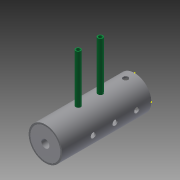
# Autodesk Inventor part: collector
Saved by Autodesk Inventor 2015 (Build 190159000, 159)
## iProperties
Created: 2014-11-05
Part Number: collector
Material: Generic
Document SubType Name: Modeling
Designer: lethcoec
Density: 1 g/cm^3
Appearance: Default
Author: lethcoec
Autodesk Inventor part; units mm, degrees
sketch "Sketch1" plane through (0, 0, 0) normal (0, 0, 1) x (1, 0, 0)
  circle A0 centre (0, 0) radius 19.05
  dimension "d0" = 38.1
  constraints: 1 centre point, 1 coincident
  measures "d0" diameter of A0
extrude "Extrusion1" add sketch "Sketch1" along normal blind 101.6
ref_plane "Work Plane1" through (19.05, 0, 0) normal (1, 0, 0) x (0, 1, 0)
sketch "Sketch3" plane through (19.05, 0, 0) normal (1, 0, 0) x (0, 1, 0)
  point P0 (0, 0)
sketch "Sketch4" plane through (19.05, 0, 0) normal (1, 0, 0) x (0, 1, 0)
  line L0 (0, 13.614358) -> (0, 19.507158)
  circle A0 centre (0, 16.560758) radius 2.9464
  point P0 (0, 0)
  dimension "d6" = 5.8928
  constraints: 2 end point, 1 midpoint, 1 vertical, 1 vertical alignment, 2 other
  measures "d6" distance of L0.start L0.end
hole "Hole1" at (19.05, 0, 16.560758) direction (-1, 0, 0) diameter 5.8928 end through all
sketch "Sketch5" plane through (19.05, 0, 0) normal (1, 0, 0) x (0, 1, 0)
  line L0 (0, 19.507155) -> (0, 38.353955)
  line L1 (0, 38.353955) -> (0, 44.246755)
  circle A0 centre (0, 41.300355) radius 2.9464
  point P0 (0, 0)
  dimension "d14" = 18.8468
  dimension "d15" = 5.8928
  constraints: 4 end point, 2 vertical, 1 midpoint, 1 vertical alignment, 2 other
  measures "d14" distance of L0.start L0.end
  measures "d15" distance of L0.end L1.end
hole "Hole2" at (19.05, 0, 41.300355) direction (-1, 0, 0) diameter 5.8928 end through all
sketch "Sketch6" plane through (19.05, 0, 0) normal (1, 0, 0) x (0, 1, 0)
  line L0 (0, 44.246748) -> (0, 63.093548)
  line L1 (0, 63.093548) -> (0, 68.986348)
  circle A0 centre (0, 66.039948) radius 2.9464
  point P0 (0, 0)
  dimension "d23" = 18.8468
  dimension "d24" = 5.8928
  constraints: 4 end point, 2 vertical, 1 midpoint, 1 vertical alignment, 2 other
  measures "d23" distance of L0.start L0.end
  measures "d24" distance of L0.end L1.end
hole "Hole3" at (19.05, 0, 66.039948) direction (-1, 0, 0) diameter 5.8928 end through all
sketch "Sketch7" plane through (0, 0, 0) normal (0, 0, -1) x (-1, 0, 0)
  circle A0 centre (0, 0) radius 19.05 projected
ref_plane "Work Plane2" through (0, 19.05, 0) normal (0, 1, 0) x (-1, 0, 0)
sketch "Sketch8" plane through (0, 19.05, 0) normal (0, 1, 0) x (-1, 0, 0)
  line L0 (0, 0) -> (0, 7.4041)
  line L1 (0, 7.4041) -> (0, 13.2969)
  circle A0 centre (0, 10.3505) radius 2.9464
  dimension "d33" = 7.4041
  dimension "d34" = 5.8928
  constraints: 4 end point, 2 vertical, 1 midpoint, 1 vertical alignment, 2 other
  measures "d33" distance of L0.start L0.end
  measures "d34" distance of L0.end L1.end
hole "Hole4" at (0, 19.05, 10.3505) direction (0, -1, 0) diameter 5.8928 end through all
sketch "Sketch9" plane through (0, 19.05, 0) normal (0, 1, 0) x (-1, 0, 0)
  line L0 (0, 13.296886) -> (0, 36.156886)
  line L1 (0, 36.156886) -> (0, 42.049686)
  circle A0 centre (0, 39.103286) radius 2.9464
  point P0 (0, 0)
  dimension "d42" = 22.86
  dimension "d43" = 5.8928
  constraints: 4 end point, 2 vertical, 1 midpoint, 1 vertical alignment, 2 other
  measures "d42" distance of L0.start L0.end
  measures "d43" distance of L0.end L1.end
sketch "Sketch10" plane through (0, 19.05, 0) normal (0, 1, 0) x (-1, 0, 0)
  line L0 (0, 42.049683) -> (0, 61.328283)
  line L1 (0, 61.328283) -> (0, 67.221083)
  circle A0 centre (0, 64.274683) radius 2.9464
  point P0 (0, 0)
  dimension "d44" = 19.2786
  dimension "d45" = 5.8928
  constraints: 4 end point, 2 vertical, 1 midpoint, 1 vertical alignment, 2 other
  measures "d44" distance of L0.start L0.end
  measures "d45" distance of L0.end L1.end
hole "Hole5" at (0, 19.05, 39.103286) direction (0, -1, 0) diameter 5.8928 end through all
hole "Hole6" at (0, 19.05, 64.274683) direction (0, -1, 0) diameter 5.8928 end through all
extrude "Extrusion2" add sketch "Sketch7" along normal blind 0.000025
sketch "Sketch11" plane through (0, 0, -0.000025) normal (0, 0, -1) x (-1, 0, 0)
  circle A0 centre (0, 0) radius 17.19707
  constraints: 1 centre point, 1 coincident
hole "Hole7" at (0, 0, -0.000025) direction (0, 0, 1) diameter 34.3916 end through all
sketch "Sketch12" plane through (0, 0, 101.6) normal (0, 0, 1) x (1, 0, 0)
  circle A0 centre (0, 0) radius 17.128601
  constraints: 1 centre point, 1 coincident
extrude "Extrusion3" add sketch "Sketch12" against normal blind 20.6883
sketch "Sketch13" plane through (0, 0, 101.6) normal (0, 0, 1) x (1, 0, 0)
  circle A0 centre (0, 0) radius 4.54787
  dimension "d72" = 9.09574
  constraints: 1 centre point, 1 coincident
  measures "d72" diameter of A0
hole "Hole8" at (0, 0, 101.6) direction (0, 0, -1) diameter 9.09574 end through all
ref_plane "Work Plane3" through (0, 19.05, 0) normal (0, 1, 0) x (-1, 0, 0)
sketch "Sketch14" plane through (0, 19.05, 0) normal (0, 1, 0) x (-1, 0, 0)
  circle A0 centre (0, 64.274694) radius 2.946394
  point P0 (0, 0)
  constraints: 1 centre point
extrude "Extrusion4" add sketch "Sketch14" along normal blind 55.2958
sketch "Sketch15" plane through (0, 74.3458, 64.274694) normal (0, 1, 0) x (1, 0, 0)
  circle A0 centre (0, 0) radius 2.00533
  point P0 (0, 64.274694)
  dimension "d82" = 4.01066
  constraints: 1 centre point
  measures "d82" diameter of A0
hole "Hole9" at (0, 74.3458, 64.274694) direction (0, -1, 0) diameter 3.99034 end through all
sketch "Sketch16" plane through (0, 19.05, 0) normal (0, -1, 0) x (1, 0, 0)
  point P0 (0, 0)
sketch "Sketch17" plane through (0, 19.05, 0) normal (0, 1, 0) x (-1, 0, 0)
  circle A0 centre (0, 39.099938) radius 2.94258
  point P0 (0, 0)
  constraints: 1 centre point
extrude "Extrusion5" add sketch "Sketch17" along normal blind 55.2958
sketch "Sketch18" plane through (0, 74.3458, 39.099938) normal (0, 1, 0) x (1, 0, 0)
  circle A0 centre (0, 0) radius 1.9939
  point P0 (0, 39.099938)
  dimension "d92" = 3.9878
  constraints: 1 centre point
  measures "d92" diameter of A0
hole "Hole10" at (0, 74.3458, 39.099938) direction (0, -1, 0) diameter 3.99034 end through all
sketch "Sketch19" plane through (0, 19.05, 39.099938) normal (0, -1, 0) x (1, 0, 0)
  circle A0 centre (0, 0) radius 2.94258
  point P0 (0, -39.099938)
  constraints: 1 centre point
extrude "Extrusion6" add sketch "Sketch19" along normal blind 18.7833
sketch "Sketch20" plane through (0, 0.2667, 39.099938) normal (0, -1, 0) x (1, 0, 0)
  circle A0 centre (0, 0) radius 1.99517
  point P0 (0, -39.099938)
  constraints: 1 centre point
hole "Hole11" at (0, 0.2667, 39.099938) direction (0, 1, 0) diameter 3.99034 end through all
sketch "Sketch21" plane through (0, 19.05, 0) normal (0, -1, 0) x (1, 0, 0)
  circle A0 centre (0, 64.264453) radius 2.9464
  point P0 (0, 0)
  dimension "d109" = 5.8928
  constraints: 1 centre point
  measures "d109" diameter of A0
extrude "Extrusion7" add sketch "Sketch21" along normal blind 18.7833
sketch "Sketch22" plane through (0, 0.2667, 64.264453) normal (0, -1, 0) x (1, 0, 0)
  circle A0 centre (0, 0) radius 1.986457
  point P0 (0, -64.264453)
  constraints: 1 centre point
hole "Hole12" at (0, 0.2667, 64.264453) direction (0, 1, 0) diameter 3.99034 end through all
body "Solid1"
